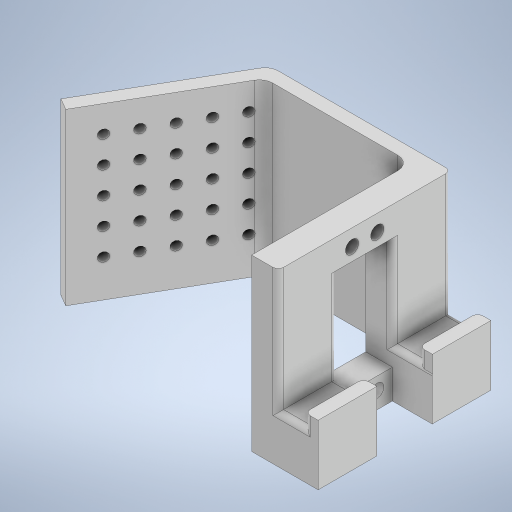
# Autodesk Inventor part: Support2
Saved by Autodesk Inventor 2024.1 (Build 281209000, 209)
## iProperties
Created: 2024-04-07
Part Number: Support2
Material: Générique
Document SubType Name: Modeling
Designer: chass
Density: 1 g/cm^3
Appearance: Par défaut
Author: chass
## iProperties of the stored document Support2_Impression 3D.ipt
Created: 2024-04-07
Part Number: Support2_Impression 3D
Material: Générique
Document SubType Name: Modeling
Designer: chass
Density: 1 g/cm^3
Appearance: Par défaut
Author: chass
Autodesk Inventor part; units mm, degrees
ref_plane "YZ Plane" through (0, 0, 0) normal (1, 0, 0) x (0, 1, 0)
ref_plane "XZ Plane" through (0, 0, 0) normal (0, 1, 0) x (-1, 0, 0)
ref_plane "XY Plane" through (0, 0, 0) normal (0, 0, 1) x (1, 0, 0)
sketch "Esquisse1" plane through (0, 0, 0) normal (1, 0, 0) x (0, 1, 0)
  line L0 (32, 32.5) -> (-32, 32.5)
  line L1 (-32, 32.5) -> (-32, -32.5)
  line L2 (-32, -32.5) -> (32, -32.5)
  line L3 (32, -32.5) -> (32, 32.5)
  line L4 (21, 10.4) -> (-21, 10.4)
  line L5 (-21, 10.4) -> (-21, -10.4)
  line L6 (-21, -10.4) -> (21, -10.4)
  line L7 (21, -10.4) -> (21, 10.4)
  line L8 (21, 10.4) -> (-21, -10.4)
  line L9 (-21, 10.4) -> (21, -10.4)
  circle A0 centre (25.791, 4.75) radius 2.5
  line L10 (32, 0) -> (21, 0)
  circle A1 centre (25.791, -4.75) radius 2.5
  line L11 (0, 10.4) -> (0, -10.4)
  circle A2 centre (-25.791, 4.75) radius 2.5
  circle A3 centre (-25.791, -4.75) radius 2.5
  point P0 (0, 0)
  point P1 (0, 0)
  point P2 (0, 0)
  point P3 (0, 0)
  point P4 (0, 0)
  dimension "d0" = 65
  dimension "d1" = 64
  dimension "d2" = 42
  dimension "d3" = 20.8
  dimension "d4" = 5
  dimension "d5" = 4.791
  dimension "d6" = 4.75
  constraints: 24 end point, 6 midpoint, 4 centre point, 4 parallel, 3 coincident, 3 symmetric about line, 2 horizontal, 2 perpendicular, 3 other
  measures "d0" distance of L2.end L0.start
  measures "d1" distance of L0.start L0.end
  measures "d2" distance of L5.end L6.end
  measures "d3" distance of L6.end L4.start
  measures "d4" diameter of A0
  measures "d5" distance from line of L7 A0.centre
  measures "d6" distance from line of L10 A0.centre
extrude "Extrusion1" add sketch "Esquisse1" along normal blind 10
sketch "Esquisse2" plane through (10, 0, 0) normal (1, 0, 0) x (0, 0, -1)
  line L0 (-10.4, -21) -> (-10.4, 21) projected
  line L1 (-32.5, -32) -> (-10.4, -32)
  line L2 (-10.4, -32) -> (-10.4, -14.325)
  line L3 (-10.4, -14.325) -> (-32.5, -14.325)
  line L4 (-32.5, -14.325) -> (-32.5, -32)
  line L5 (0, -32) -> (0, 32)
  line L6 (32.5, -32) -> (-32.5, -32)
  line L7 (10.4, -32) -> (10.4, -14.325)
  line L8 (10.4, -14.325) -> (32.5, -14.325)
  line L9 (32.5, -14.325) -> (32.5, -32)
  point P0 (0, 0)
  dimension "d9" = 17.675
  constraints: 18 end point, 5 symmetric about line, 2 parallel, 1 horizontal, 1 perpendicular, 1 point on line, 1 vertical
  measures "d9" distance of L2.end L1.end
extrude "Extrusion2" add sketch "Esquisse2" along normal blind 15
sketch "Esquisse3" plane through (10, -14.325, 32.5) normal (0, 1, 0) x (1, 0, 0)
  line L0 (15, 22.1) -> (15, 0) projected
  line L1 (0, 22.1) -> (15, 22.1) projected
  line L2 (15, 0) -> (10, 0)
  line L3 (10, 0) -> (10, 22.1)
  line L4 (10, 22.1) -> (15, 22.1)
  line L5 (15, 22.1) -> (15, 0)
  line L6 (-10, 65) -> (15, 65) projected
  line L7 (15, 43) -> (10, 43)
  line L8 (10, 43) -> (10, 65)
  line L9 (10, 65) -> (15, 65)
  line L10 (15, 65) -> (15, 43)
  point P0 (-10, 32.5)
  constraints: 16 end point, 4 parallel, 4 point on line, 2 horizontal, 2 perpendicular
extrude "Extrusion3" add sketch "Esquisse3" along normal blind 5
sketch "Esquisse4" plane through (0, 0, 0) normal (-1, 0, 0) x (0, 0, 1)
  line L0 (-32.5, -32) -> (-32.5, 32) projected
  line L1 (32.5, -32) -> (-32.5, -32) projected
  line L2 (-32.5, 32) -> (-27.5, 32)
  line L3 (-27.5, 32) -> (-27.5, -32)
  line L4 (-27.5, -32) -> (-32.5, -32)
  line L5 (-32.5, -32) -> (-32.5, 32)
  point P0 (0, 0)
  dimension "d14" = 5
  constraints: 8 end point, 2 parallel, 1 horizontal, 1 perpendicular, 1 point on line
  measures "d14" distance of L3.end L4.end
extrude "Extrusion4" add sketch "Esquisse4" along normal blind 55
sketch "Esquisse5" plane through (0, 32, 32.5) normal (0, 1, 0) x (1, 0, 0)
  line L0 (0, 60) -> (-55, 60) projected
  line L1 (-55, 60) -> (-82.4241, 12.5)
  line L2 (-55, 60) -> (-0.1517, 60) construction
  line L3 (-82.4241, 12.5) -> (-86.7543, 15)
  line L4 (-86.7543, 15) -> (-57.8868, 65)
  line L5 (-55, 65) -> (25, 65) projected
  line L6 (-57.8868, 65) -> (-55, 65)
  line L7 (-55, 60) -> (-55, 65)
  point P0 (0, 32.5)
  dimension "d17" = 120
  dimension "d18" = 5
  dimension "d19" = 90
  dimension "d53" = 50
  constraints: 12 end point, 2 horizontal, 2 perpendicular, 1 equal length
  measures "d17" angle of L1 L2
  measures "d18" distance of L1.end L3.end
  measures "d19" angle of L3 L4
  measures "d53" vertical distance of L3.end L4.end
extrude "Extrusion5" add sketch "Esquisse5" against normal blind 64
sketch "Esquisse6" plane through (-57.8868, -32, -32.5) normal (-0.8660254, 0, -0.5) x (-0.5, 0, 0.8660254)
  circle A0 centre (7.3483, 54) radius 1.75
  line L0 (7.3483, 54) -> (17.3483, 54)
  circle A1 centre (17.3483, 54) radius 1.75
  line L1 (17.3483, 54) -> (27.3483, 54)
  circle A2 centre (27.3483, 54) radius 1.75
  line L2 (0, 64) -> (0, 0) projected
  line L3 (56, 0) -> (0, 0)
  line L4 (27.3483, 64) -> (27.3483, 0) projected
  line L5 (27.3483, 0) -> (27.3483, 64)
  circle A3 centre (47.3483, 54) radius 1.75
  circle A4 centre (37.3483, 54) radius 1.75
  line L6 (5.5983, 49) -> (49.0983, 49)
  line L7 (5.5983, 49) -> (49.0983, 49) construction
  circle A5 centre (7.3483, 44) radius 1.75
  circle A6 centre (17.3483, 44) radius 1.75
  circle A7 centre (27.3483, 44) radius 1.75
  circle A8 centre (47.3483, 44) radius 1.75
  circle A9 centre (37.3483, 44) radius 1.75
  line L8 (5.5983, 39) -> (49.0983, 39)
  circle A10 centre (7.3483, 24) radius 1.75
  line L9 (7.3483, 24) -> (17.3483, 24)
  circle A11 centre (17.3483, 24) radius 1.75
  line L10 (17.3483, 24) -> (27.3483, 24)
  circle A12 centre (27.3483, 24) radius 1.75
  circle A13 centre (47.3483, 24) radius 1.75
  circle A14 centre (37.3483, 24) radius 1.75
  line L11 (5.5983, 29) -> (49.0983, 29)
  line L12 (5.5983, 29) -> (49.0983, 29) construction
  circle A15 centre (7.3483, 34) radius 1.75
  circle A16 centre (17.3483, 34) radius 1.75
  circle A17 centre (27.3483, 34) radius 1.75
  circle A18 centre (37.3483, 34) radius 1.75
  circle A19 centre (47.3483, 34) radius 1.75
  line L13 (5.5983, 19) -> (49.0983, 19)
  circle A20 centre (27.3483, 14) radius 1.75
  line L14 (17.3483, 14) -> (27.3483, 14)
  line L15 (7.3483, 14) -> (17.3483, 14)
  circle A21 centre (7.3483, 14) radius 1.75
  circle A22 centre (17.3483, 14) radius 1.75
  circle A23 centre (37.3483, 14) radius 1.75
  circle A24 centre (47.3483, 14) radius 1.75
  line L16 (0, 64) -> (57.735, 64) projected
  dimension "d41" = 3.5
  dimension "d42" = 3.5
  dimension "d43" = 10
  dimension "d44" = 10
  dimension "d45" = 3.5
  dimension "d47" = 5
  dimension "d48" = 5
  dimension "d49" = 5
  constraints: 29 symmetric about line, 28 end point, 25 centre point, 6 coincident, 5 horizontal, 2 collinear, 1 perpendicular, 1 point on line, 22 other
  measures "d41" diameter of A0
  measures "d42" diameter of A1
  measures "d43" distance of L0.start L0.end
  measures "d44" distance of L1.start L1.end
  measures "d45" diameter of A2
  measures "d47" distance from line of L6 L1.end
  measures "d48" distance from line of L8 A7.centre
  measures "d49" distance from line of L13 A12.centre
extrude "Extrusion6" cut sketch "Esquisse6" against normal blind 10 contours A0 | A1 L1 L0 | L0 L1 A1 | A2 L4 L1 | L1 L4 A2 | L4 A2 | A7 L4 | L4 A7 | A20 L14 L4 | L4 A20 | A17 L4 | L4 A17 | L14 A20 L4 | A12 L4 | L4 L10 A12 | A12 L10 L4 | A3 | A4 | A5 | A6 | A8 | A9 | A10 | A11 L10 L9 | L9 L10 A11 | A13 | A14 | A15 | A16 | A18 | A19 | L15 A22 L14 | L14 A22 L15 | A21 | A23 | A24
fillet "Congé de faces1" radius 5 1 edges at (-55, 0, -27.5)
fillet "Congé de faces2" radius 5 1 edges at (0, 0, -27.5)
fillet "Congé1" radius 2 8 edges at (20, -11.825, -10.5) (10, 3.3375, -10.4) (10, 3.3375, 10.4) (20, -11.825, 10.4) (10, 8.8375, 32.5) (20, -11.825, 32.5) (10, 8.8375, -32.5) (20, -11.825, -32.5)
fillet "Congé2" radius 2 4 edges at (9, -14.325, -10.4) (17.5, -14.325, -10.4) (9, -14.325, 10.4) (21, -14.325, 10.4)
fillet "Congé3" radius 2 4 edges at (21, -14.325, 32.5) (9, -14.325, 32.5) (21, -14.325, -32.5) (9, -14.325, -32.5)
fillet "Congé de faces3" radius 5 1 edges at (-57.8868, 0, -32.5)
